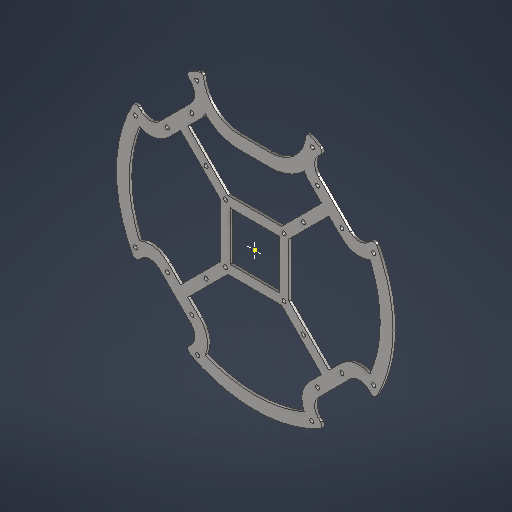
# Autodesk Inventor part: Mittelding mit IR Halterung
Saved by Autodesk Inventor 2025.3 (Build 293356000, 356)
## iProperties
Created: 2024-10-04
Part Number: Mittelding mit IR Halterung
Material: Generisch
Document SubType Name: Modeling
Designer: Mathimazierer
Density: 1 g/cm^3
Appearance: Halbpoliert
Author: Mathimazierer
Autodesk Inventor part; units mm, degrees
ref_plane "YZ Plane" through (0, 0, 0) normal (1, 0, 0) x (0, 1, 0)
ref_plane "XZ Plane" through (0, 0, 0) normal (0, 1, 0) x (-1, 0, 0)
ref_plane "XY Plane" through (0, 0, 0) normal (0, 0, 1) x (1, 0, 0)
sketch "Skizze1" plane through (0, 0, 0) normal (0, 1, 0) x (-1, 0, 0)
  circle A0 centre (48.7904, 67.8822) radius 1.6
  circle A1 centre (48.7904, -67.8823) radius 1.6
  circle A2 centre (-48.7904, -67.8822) radius 1.6
  circle A3 centre (-48.7904, 67.8823) radius 1.6
  circle A4 centre (67.8823, 48.7904) radius 1.6
  circle A5 centre (67.8822, -48.7904) radius 1.6
  circle A6 centre (-67.8823, -48.7904) radius 1.6
  circle A7 centre (-67.8822, 48.7904) radius 1.6
  arc A8 (42.6492, 98.6778) -> (39.8653, 97.0378) centre (41.8557, 96.8419) ccw
  arc A9 (12, 71.781) -> (39.8653, 97.0378) centre (12, 99.781) ccw
  line L0 (-12, 71.781) -> (12, 71.781)
  arc A10 (-39.8653, 97.0378) -> (-12, 71.781) centre (-12, 99.781) ccw
  arc A11 (-39.8653, 97.0378) -> (-42.6492, 98.6778) centre (-41.8557, 96.8419) ccw
  arc A12 (-42.6492, 98.6778) -> (-50.5184, 94.8902) centre (0, 0) ccw
  arc A13 (-50.5184, 94.8902) -> (-51.2299, 90.1208) centre (-49.1086, 92.2421) ccw
  line L1 (-49.4975, 88.3883) -> (-51.2299, 90.1208)
  arc A14 (-49.4975, 74.2462) -> (-49.4975, 88.3883) centre (-56.5685, 81.3173) ccw
  line L2 (-74.2462, 49.4975) -> (-49.4975, 74.2462)
  arc A15 (-88.3883, 49.4975) -> (-74.2462, 49.4975) centre (-81.3173, 56.5685) ccw
  line L3 (-90.1207, 51.2299) -> (-88.3883, 49.4975)
  arc A16 (-90.1207, 51.2299) -> (-94.8902, 50.5184) centre (-92.2421, 49.1086) ccw
  arc A17 (-94.8902, 50.5184) -> (-94.8902, -50.5184) centre (0, 0) ccw
  arc A18 (-94.8902, -50.5184) -> (-90.1208, -51.2299) centre (-92.2421, -49.1086) ccw
  line L4 (-88.3883, -49.4975) -> (-90.1208, -51.2299)
  arc A19 (-74.2462, -49.4975) -> (-88.3883, -49.4975) centre (-81.3173, -56.5685) ccw
  line L5 (-49.4975, -74.2462) -> (-74.2462, -49.4975)
  arc A20 (-49.4975, -88.3883) -> (-49.4975, -74.2462) centre (-56.5685, -81.3173) ccw
  line L6 (-51.2299, -90.1207) -> (-49.4975, -88.3883)
  arc A21 (-51.2299, -90.1207) -> (-50.5184, -94.8902) centre (-49.1086, -92.2421) ccw
  arc A22 (-50.5184, -94.8902) -> (50.5184, -94.8902) centre (0, 0) ccw
  arc A23 (50.5184, -94.8902) -> (51.2299, -90.1208) centre (49.1086, -92.2421) ccw
  line L7 (49.4975, -88.3883) -> (51.2299, -90.1208)
  arc A24 (49.4975, -74.2462) -> (49.4975, -88.3883) centre (56.5685, -81.3173) ccw
  line L8 (74.2462, -49.4975) -> (49.4975, -74.2462)
  arc A25 (88.3883, -49.4975) -> (74.2462, -49.4975) centre (81.3173, -56.5685) ccw
  line L9 (90.1207, -51.2299) -> (88.3883, -49.4975)
  arc A26 (90.1207, -51.2299) -> (94.8902, -50.5184) centre (92.2421, -49.1086) ccw
  arc A27 (94.8902, -50.5184) -> (94.8902, 50.5184) centre (0, 0) ccw
  arc A28 (94.8902, 50.5184) -> (90.1208, 51.2299) centre (92.2421, 49.1086) ccw
  line L10 (88.3883, 49.4975) -> (90.1208, 51.2299)
  arc A29 (74.2462, 49.4975) -> (88.3883, 49.4975) centre (81.3173, 56.5685) ccw
  line L11 (49.4975, 74.2462) -> (74.2462, 49.4975)
  arc A30 (49.4975, 88.3883) -> (49.4975, 74.2462) centre (56.5685, 81.3173) ccw
  line L12 (51.2299, 90.1207) -> (49.4975, 88.3883)
  arc A31 (51.2299, 90.1207) -> (50.5184, 94.8902) centre (49.1086, 92.2421) ccw
  arc A32 (50.5184, 94.8902) -> (42.6492, 98.6778) centre (0, 0) ccw
  line L13 (-107.5, 0) -> (-97.5, 0)
  circle A33 centre (0, 0) radius 97.5
  line L14 (0, 71.781) -> (0, 61.781)
  line L15 (-12, 99.781) -> (12, 99.781) construction
  line L16 (-12, 137.781) -> (12, 137.781)
  line L17 (12, 61.781) -> (-12, 61.781)
  arc A34 (-12, 137.781) -> (-12, 61.781) centre (-12, 99.781) ccw
  arc A35 (12, 61.781) -> (12, 137.781) centre (12, 99.781) ccw
  circle A36 centre (0, 0) radius 107.5
  line L18 (61.8718, 61.8718) -> (54.8008, 54.8008)
  line L19 (56.5685, 81.3173) -> (81.3173, 56.5685) construction
  line L20 (70.7107, 95.4594) -> (95.4594, 70.7107)
  line L21 (67.1751, 42.4264) -> (42.4264, 67.1751)
  arc A37 (70.7107, 95.4594) -> (42.4264, 67.1751) centre (56.5685, 81.3173) ccw
  arc A38 (67.1751, 42.4264) -> (95.4594, 70.7107) centre (81.3173, 56.5685) ccw
  line L22 (-95.4594, 70.7107) -> (-70.7107, 95.4594)
  arc A39 (-95.4594, 70.7107) -> (-67.1751, 42.4264) centre (-81.3173, 56.5685) ccw
  line L23 (-42.4264, 67.1751) -> (-67.1751, 42.4264)
  arc A40 (-42.4264, 67.1751) -> (-70.7107, 95.4594) centre (-56.5685, 81.3173) ccw
  line L24 (-70.7107, -95.4594) -> (-95.4594, -70.7107)
  arc A41 (-70.7107, -95.4594) -> (-42.4264, -67.1751) centre (-56.5685, -81.3173) ccw
  line L25 (-67.1751, -42.4264) -> (-42.4264, -67.1751)
  arc A42 (-67.1751, -42.4264) -> (-95.4594, -70.7107) centre (-81.3173, -56.5685) ccw
  line L26 (95.4594, -70.7107) -> (70.7107, -95.4594)
  arc A43 (95.4594, -70.7107) -> (67.1751, -42.4264) centre (81.3173, -56.5685) ccw
  line L27 (42.4264, -67.1751) -> (67.1751, -42.4264)
  arc A44 (42.4264, -67.1751) -> (70.7107, -95.4594) centre (56.5685, -81.3173) ccw
  point P0 (0, 0)
  point P1 (0, 99.781)
  point P2 (68.9429, 68.9429)
  point P3 (38.5642, 72.6085)
  point P4 (89.6293, 38.3776)
  point P5 (89.6293, -38.3776)
  point P6 (38.3776, -89.6293)
  point P7 (-38.3776, -89.6293)
  point P8 (-89.6293, -38.3776)
  point P9 (-89.6293, 38.3776)
  point P10 (-38.5642, 72.6085)
  dimension "d2" = 10
  dimension "d3" = 10
  dimension "d4" = 10
  dimension "d5" = 360
  constraints: 71 point on circle, 60 end point, 44 centre point, 8 tangent, 4 midpoint, 2 horizontal, 2 parallel, 1 coincident, 1 concentric, 1 vertical, 44 other
  measures "d2" distance of L13.start L13.end
  measures "d3" distance of L14.start L14.end
  measures "d4" distance of L18.start L18.end
extrude "Extrusion1" add sketch "Skizze1" along normal blind 2 contours A32 A37 A33 A9 A8 | A32 A35 A33 A37 | A11 A10 A33 A40 A12 | A33 A37 A35 L17 L14 L0 A9 | A32 A31 L12 A30 A33 A35 | A33 A35 A37 | A40 A33 A34 A12 | A10 L0 L14 L17 A34 A40 A33 | A33 A30 L11 L18 L21 A37 A35 | A34 A33 A14 L1 A13 A12 | A40 A34 A33 | A27 A38 A33 A29 L10 A28 | A34 A40 L23 A39 A33 A15 L2 A14 | A27 A43 A33 A38 | A33 A38 L21 L18 L11 A29 | A16 L3 A15 A33 A39 A17 | A39 A33 L13 A17 | A27 A26 L9 A25 A33 A43 | L13 A33 A42 A17 | A33 A25 L8 A24 A44 L27 A43 | A42 A33 A19 L4 A18 A17 | A22 A44 A33 A24 L7 A23 | A42 L25 A41 A33 A20 L5 A19 | A22 A41 A33 A44 | A21 L6 A20 A33 A41 A22
sketch "Skizze2" plane through (0, 0, 0) normal (0, -1, 0) x (1, 0, 0)
  line L0 (-12, 71.781) -> (12, 71.781)
  line L1 (0, 71.781) -> (-45, 71.781)
  line L2 (-45, 71.781) -> (-45, 90.181)
  circle A0 centre (-45, 91.781) radius 1.6
  circle A1 centre (45, 91.781) radius 1.6
  line L3 (-45, 91.781) -> (-43.4, 91.781)
  line L4 (43.4, 91.781) -> (45, 91.781)
  point P0 (0, 0)
  point P1 (0, 0)
  dimension "d12" = 3.2
  dimension "d8" = 45
  dimension "d9" = 20
  dimension "d10" = 90
  dimension "d11" = 3.2
  constraints: 10 end point, 3 perpendicular, 2 coincident, 2 point on circle, 1 centre point, 1 collinear, 1 horizontal alignment, 1 midpoint, 2 other
  measures "d8" distance of L1.start L1.end
  measures "d9" distance of L1.end L3.start
  measures "d10" distance of L3.start L4.end
  measures "d11" diameter of A0
extrude "Extrusion2" cut sketch "Skizze2" against normal blind 2
sketch "Skizze4" plane through (0, 0, 0) normal (0, -1, 0) x (1, 0, 0)
  arc A0 (-89.6293, 38.3776) -> (-67.1751, 42.4264) centre (-81.3173, 56.5685) ccw projected
  line L0 (-89.6293, 38.3776) -> (-92.6293, 38.3776)
  line L1 (-92.6293, 38.3776) -> (-92.6293, 44.3776)
  circle A1 centre (-92.6293, 44.3776) radius 1.6
  line L2 (0, 0) -> (0, 25.0605)
  circle A2 centre (92.6293, 44.3776) radius 1.6
  line L3 (0, 0) -> (24.0144, 0)
  circle A3 centre (-92.6293, -44.3776) radius 1.6
  circle A4 centre (92.6293, -44.3776) radius 1.6
  circle A5 centre (-44.3776, -92.6293) radius 1.6
  circle A6 centre (44.3776, -92.6293) radius 1.6
  point P0 (0, 0)
  dimension "d15" = 3
  dimension "d16" = 6
  dimension "d17" = 3.2
  dimension "d18" = 3.2
  constraints: 8 end point, 6 centre point, 3 symmetric about line, 2 horizontal, 1 coincident, 1 perpendicular, 1 vertical, 3 other
  measures "d15" distance of L0.start L0.end
  measures "d16" distance of L0.end L1.end
  measures "d17" diameter of A1
  measures "d18" diameter of A5
extrude "Extrusion3" cut sketch "Skizze4" against normal blind 3.2
sketch "Skizze5" plane through (0, 0, 0) normal (0, -1, 0) x (1, 0, 0)
  line L0 (-42.4264, 67.1751) -> (-67.1751, 42.4264) projected
  line L1 (-54.8008, 54.8008) -> (-14.8008, 54.8008) construction
  line L2 (-54.8008, 54.8008) -> (-26.5165, 26.5165)
  line L3 (-54.8008, -54.8008) -> (-26.5165, -26.5165)
  line L4 (54.8008, -54.8008) -> (26.5165, -26.5165)
  line L5 (54.8008, 54.8008) -> (26.5165, 26.5165)
  line L6 (-26.5165, 26.5165) -> (-26.5165, -26.5165)
  line L7 (26.5165, -26.5165) -> (-26.5165, -26.5165)
  line L8 (26.5165, -26.5165) -> (26.5165, 26.5165)
  line L9 (-26.5165, 26.5165) -> (26.5165, 26.5165)
  line L10 (-54.8008, 54.8008) -> (-57.6292, 51.9723)
  line L11 (-57.6292, 51.9723) -> (-51.9724, 57.6292)
  line L12 (-51.9724, 57.6292) -> (-20.8597, 26.5165)
  line L13 (-57.6292, 51.9723) -> (-26.5165, 20.8596)
  line L14 (-57.6292, -51.9724) -> (-26.5165, -20.8597)
  line L15 (-51.9723, -57.6292) -> (-20.8596, -26.5165)
  line L16 (51.9724, -57.6292) -> (20.8597, -26.5165)
  line L17 (57.6292, -51.9723) -> (26.5165, -20.8596)
  line L18 (57.6292, 51.9724) -> (26.5165, 20.8597)
  line L19 (51.9723, 57.6292) -> (20.8596, 26.5165)
  line L20 (51.9723, 57.6292) -> (57.6292, 51.9724)
  line L21 (51.9724, -57.6292) -> (57.6292, -51.9723)
  line L22 (-57.6292, -51.9724) -> (-51.9723, -57.6292)
  line L23 (-67.1751, -42.4264) -> (-42.4264, -67.1751) projected
  line L24 (-26.5165, 26.5165) -> (-26.5165, 19.0165)
  line L25 (-26.5165, 19.0165) -> (-19.0165, 19.0165)
  line L26 (26.5165, -26.5165) -> (19.0165, -26.5165)
  line L27 (19.0165, -26.5165) -> (19.0165, -19.0165)
  line L28 (-19.0165, 19.0165) -> (19.0165, 19.0165)
  line L29 (19.0165, 19.0165) -> (19.0165, -19.0165)
  line L30 (19.0165, -19.0165) -> (-19.0165, -19.0165)
  line L31 (-19.0165, -19.0165) -> (-19.0165, 19.0165)
  circle A0 centre (-22.7665, 22.7665) radius 1.6
  circle A1 centre (22.7665, 22.7665) radius 1.6
  circle A2 centre (-22.7665, -22.7665) radius 1.6
  circle A3 centre (22.7665, -22.7665) radius 1.6
  line L32 (-26.5165, 20.8596) -> (-40.6586, 35.0018)
  line L33 (-40.6586, 35.0018) -> (-37.8302, 37.8302)
  circle A4 centre (-37.8302, 37.8302) radius 1.65
  circle A5 centre (-37.8302, -37.8302) radius 1.65
  circle A6 centre (37.8302, -37.8302) radius 1.65
  circle A7 centre (37.8302, 37.8302) radius 1.65
  point P0 (0, 0)
  point P1 (-26.5165, -20.8597)
  point P2 (20.8597, -26.5165)
  point P3 (26.5165, 20.8597)
  dimension "d23" = 40
  dimension "d26" = 360
  dimension "d28" = 4
  dimension "d29" = 8
  dimension "d32" = 360
  dimension "d34" = 7.5
  dimension "d35" = 7.5
  dimension "d36" = 7.5
  dimension "d37" = 7.5
  dimension "d38" = 3.2
  dimension "d39" = 3.2
  dimension "d40" = 3.2
  dimension "d41" = 3.2
  dimension "d44" = 20
  dimension "d45" = 3.3
  dimension "d48" = 360
  constraints: 64 end point, 10 perpendicular, 8 centre point, 8 point on line, 3 parallel, 2 horizontal, 1 coincident, 1 collinear, 1 midpoint, 1 vertical, 47 other
  measures "d23" distance of L1.start L2.end
  measures "d28" distance of L1.start L10.end
  measures "d29" distance of L10.end L11.end
  measures "d34" distance of L2.end L24.end
  measures "d35" distance of L24.end L25.end
  measures "d36" distance of L4.end L26.end
  measures "d37" distance of L26.end L27.end
  measures "d38" diameter of A0
  measures "d39" diameter of A1
  measures "d40" diameter of A2
  measures "d41" diameter of A3
  measures "d44" distance of L13.end L32.end
  measures "d45" diameter of A4
extrude "Extrusion4" add sketch "Skizze5" against normal blind 2 contours L12 L9 L2 A4 L0 | L2 A4 L33 L13 L0 | L9 L8 L7 L27 L29 L28 L25 L6 | A4 L2 | L2 L33 A4 | L6 L13 L33 A4 L2 | L19 L20 L5 A7 L9 | L2 A4 L33 | L5 A7 L20 L18 L8 | L25 L31 L30 L27 L7 L6 | A7 L5 | L5 A7 | L6 L3 A5 L22 L14 | L17 L21 L4 A6 L8 | L7 L15 L22 L3 A5 | L4 A6 L21 L16 L7 | A5 L3 | L3 A5 | A6 L4 | L4 A6
sketch "Skizze6" plane through (0, 2, 0) normal (0, 1, 0) x (1, 0, 0)
  line L0 (-51.9723, 57.6292) -> (-42.4264, 67.1751) projected
  arc A0 (-42.4264, 67.1751) -> (-38.3776, 89.6293) centre (-56.5685, 81.3173) ccw projected
  arc A1 (38.3776, 89.6293) -> (-38.3776, 89.6293) centre (0, 0) ccw projected
  arc A2 (38.3776, 89.6293) -> (42.4264, 67.1751) centre (56.5685, 81.3173) ccw projected
  line L1 (42.4264, 67.1751) -> (51.9724, 57.6292) projected
  line L2 (51.9724, 57.6292) -> (20.8597, 26.5165) projected
  line L3 (20.8597, 26.5165) -> (-20.8596, 26.5165) projected
  line L4 (-20.8596, 26.5165) -> (-51.9723, 57.6292) projected
  line L5 (57.6292, 51.9723) -> (67.1751, 42.4264) projected
  arc A3 (67.1751, 42.4264) -> (89.6293, 38.3776) centre (81.3173, 56.5685) ccw projected
  arc A4 (89.6293, -38.3776) -> (89.6293, 38.3776) centre (0, 0) ccw projected
  arc A5 (89.6293, -38.3776) -> (67.1751, -42.4264) centre (81.3173, -56.5685) ccw projected
  line L6 (67.1751, -42.4264) -> (57.6292, -51.9724) projected
  line L7 (57.6292, -51.9724) -> (26.5165, -20.8597) projected
  line L8 (26.5165, -20.8597) -> (26.5165, 20.8596) projected
  line L9 (26.5165, 20.8596) -> (57.6292, 51.9723) projected
  line L10 (51.9723, -57.6292) -> (42.4264, -67.1751) projected
  arc A6 (42.4264, -67.1751) -> (38.5642, -72.6085) centre (56.5685, -81.3173) ccw projected
  arc A7 (38.5642, -72.6085) -> (12, -61.781) centre (12, -99.781) ccw projected
  line L11 (12, -61.781) -> (-12, -61.781) projected
  arc A8 (-12, -61.781) -> (-38.5642, -72.6085) centre (-12, -99.781) ccw projected
  arc A9 (-38.5642, -72.6085) -> (-42.4264, -67.1751) centre (-56.5685, -81.3173) ccw projected
  line L12 (-42.4264, -67.1751) -> (-51.9724, -57.6292) projected
  line L13 (-51.9724, -57.6292) -> (-20.8597, -26.5165) projected
  line L14 (-20.8597, -26.5165) -> (20.8596, -26.5165) projected
  line L15 (20.8596, -26.5165) -> (51.9723, -57.6292) projected
  circle A10 centre (-22.7665, -22.7665) radius 1.6 projected
  circle A11 centre (22.7665, -22.7665) radius 1.6 projected
  circle A12 centre (22.7665, 22.7665) radius 1.6 projected
  circle A13 centre (-22.7665, 22.7665) radius 1.6 projected
  line L16 (19.0165, -19.0165) -> (-19.0165, -19.0165) projected
  line L17 (-19.0165, -19.0165) -> (-19.0165, 19.0165) projected
  line L18 (-19.0165, 19.0165) -> (19.0165, 19.0165) projected
  line L19 (19.0165, 19.0165) -> (19.0165, -19.0165) projected
  circle A14 centre (-44.3776, 92.6293) radius 1.6 projected
  circle A15 centre (92.6293, -44.3776) radius 1.6 projected
  circle A16 centre (-92.6293, 44.3776) radius 1.6 projected
  circle A17 centre (44.3776, 92.6293) radius 1.6 projected
  circle A18 centre (92.6293, 44.3776) radius 1.6 projected
  circle A19 centre (-92.6293, -44.3776) radius 1.6 projected
  circle A20 centre (45, -91.781) radius 1.6 projected
  circle A21 centre (-45, -91.781) radius 1.6 projected
  arc A22 (39.8653, -97.0378) -> (12, -71.781) centre (12, -99.781) ccw projected
  arc A23 (39.8653, -97.0378) -> (42.6492, -98.6778) centre (41.8557, -96.8419) ccw projected
  arc A24 (42.6492, -98.6778) -> (50.5184, -94.8902) centre (0, 0) ccw projected
  arc A25 (50.5184, -94.8902) -> (51.2299, -90.1208) centre (49.1086, -92.2421) ccw projected
  line L20 (51.2299, -90.1208) -> (49.4975, -88.3883) projected
  arc A26 (49.4975, -74.2462) -> (49.4975, -88.3883) centre (56.5685, -81.3173) ccw projected
  line L21 (49.4975, -74.2462) -> (74.2462, -49.4975) projected
  arc A27 (88.3883, -49.4975) -> (74.2462, -49.4975) centre (81.3173, -56.5685) ccw projected
  line L22 (88.3883, -49.4975) -> (90.1207, -51.2299) projected
  arc A28 (90.1207, -51.2299) -> (94.8902, -50.5184) centre (92.2421, -49.1086) ccw projected
  arc A29 (94.8902, -50.5184) -> (94.8902, 50.5184) centre (0, 0) ccw projected
  arc A30 (94.8902, 50.5184) -> (90.1208, 51.2299) centre (92.2421, 49.1086) ccw projected
  line L23 (90.1208, 51.2299) -> (88.3883, 49.4975) projected
  arc A31 (74.2462, 49.4975) -> (88.3883, 49.4975) centre (81.3173, 56.5685) ccw projected
  line L24 (74.2462, 49.4975) -> (49.4975, 74.2462) projected
  arc A32 (49.4975, 88.3883) -> (49.4975, 74.2462) centre (56.5685, 81.3173) ccw projected
  line L25 (49.4975, 88.3883) -> (51.2299, 90.1207) projected
  arc A33 (51.2299, 90.1207) -> (50.5184, 94.8902) centre (49.1086, 92.2421) ccw projected
  arc A34 (50.5184, 94.8902) -> (-50.5184, 94.8902) centre (0, 0) ccw projected
  arc A35 (-50.5184, 94.8902) -> (-51.2299, 90.1208) centre (-49.1086, 92.2421) ccw projected
  line L26 (-51.2299, 90.1208) -> (-49.4975, 88.3883) projected
  arc A36 (-49.4975, 74.2462) -> (-49.4975, 88.3883) centre (-56.5685, 81.3173) ccw projected
  line L27 (-49.4975, 74.2462) -> (-74.2462, 49.4975) projected
  arc A37 (-88.3883, 49.4975) -> (-74.2462, 49.4975) centre (-81.3173, 56.5685) ccw projected
  line L28 (-88.3883, 49.4975) -> (-90.1207, 51.2299) projected
  arc A38 (-90.1207, 51.2299) -> (-94.8902, 50.5184) centre (-92.2421, 49.1086) ccw projected
  arc A39 (-94.8902, 50.5184) -> (-94.8902, -50.5184) centre (0, 0) ccw projected
  arc A40 (-94.8902, -50.5184) -> (-90.1208, -51.2299) centre (-92.2421, -49.1086) ccw projected
  line L29 (-90.1208, -51.2299) -> (-88.3883, -49.4975) projected
  arc A41 (-74.2462, -49.4975) -> (-88.3883, -49.4975) centre (-81.3173, -56.5685) ccw projected
  line L30 (-74.2462, -49.4975) -> (-49.4975, -74.2462) projected
  arc A42 (-49.4975, -88.3883) -> (-49.4975, -74.2462) centre (-56.5685, -81.3173) ccw projected
  line L31 (-49.4975, -88.3883) -> (-51.2299, -90.1207) projected
  arc A43 (-51.2299, -90.1207) -> (-50.5184, -94.8902) centre (-49.1086, -92.2421) ccw projected
  arc A44 (-50.5184, -94.8902) -> (-42.6492, -98.6778) centre (0, 0) ccw projected
  arc A45 (-42.6492, -98.6778) -> (-39.8653, -97.0378) centre (-41.8557, -96.8419) ccw projected
  arc A46 (-12, -71.781) -> (-39.8653, -97.0378) centre (-12, -99.781) ccw projected
  line L32 (-12, -71.781) -> (12, -71.781) projected
  line L33 (-57.6292, 51.9724) -> (-26.5165, 20.8597) projected
  line L34 (-26.5165, 20.8597) -> (-26.5165, -20.8596) projected
  line L35 (-26.5165, -20.8596) -> (-57.6292, -51.9723) projected
  line L36 (-57.6292, -51.9723) -> (-67.1751, -42.4264) projected
  arc A47 (-67.1751, -42.4264) -> (-89.6293, -38.3776) centre (-81.3173, -56.5685) ccw projected
  arc A48 (-89.6293, 38.3776) -> (-89.6293, -38.3776) centre (0, 0) ccw projected
  arc A49 (-89.6293, 38.3776) -> (-67.1751, 42.4264) centre (-81.3173, 56.5685) ccw projected
  line L37 (-67.1751, 42.4264) -> (-57.6292, 51.9724) projected
  circle A50 centre (-48.7904, -67.8822) radius 1.6 projected
  circle A51 centre (48.7904, -67.8823) radius 1.6 projected
  circle A52 centre (67.8822, -48.7904) radius 1.6 projected
  circle A53 centre (-67.8823, -48.7904) radius 1.6 projected
  circle A54 centre (67.8823, 48.7904) radius 1.6 projected
  circle A55 centre (48.7904, 67.8822) radius 1.6 projected
  circle A56 centre (-48.7904, 67.8823) radius 1.6 projected
  circle A57 centre (-67.8822, 48.7904) radius 1.6 projected
sketch "Skizze8" plane through (0, 0, 0) normal (0, -1, 0) x (1, 0, 0)
  line L0 (-314.1721, 98.2713) -> (-338.9208, 73.5225)
  line L1 (-326.5464, 85.8969) -> (-286.5464, 85.8969) construction
  line L2 (-326.5464, 85.8969) -> (-298.2622, 57.6126)
  line L3 (-326.5464, -23.7046) -> (-298.2622, 4.5796)
  line L4 (-216.9449, -23.7046) -> (-245.2292, 4.5796)
  line L5 (-216.9449, 85.8969) -> (-245.2292, 57.6126)
  line L6 (-298.2622, 57.6126) -> (-298.2622, 4.5796)
  line L7 (-245.2292, 4.5796) -> (-298.2622, 4.5796)
  line L8 (-245.2292, 4.5796) -> (-245.2292, 57.6126)
  line L9 (-298.2622, 57.6126) -> (-245.2292, 57.6126)
  line L10 (-326.5464, 85.8969) -> (-329.3749, 83.0685)
  line L11 (-329.3749, 83.0685) -> (-323.718, 88.7253)
  line L12 (-323.718, 88.7253) -> (-292.6053, 57.6126)
  line L13 (-329.3749, 83.0685) -> (-298.2622, 51.9558)
  line L14 (-329.3749, -20.8762) -> (-298.2622, 10.2365)
  line L15 (-323.718, -26.5331) -> (-292.6053, 4.5796)
  line L16 (-219.7733, -26.5331) -> (-250.886, 4.5796)
  line L17 (-214.1165, -20.8762) -> (-245.2292, 10.2365)
  line L18 (-214.1165, 83.0685) -> (-245.2292, 51.9558)
  line L19 (-219.7733, 88.7253) -> (-250.886, 57.6126)
  line L20 (-329.3749, -20.8762) -> (-323.718, -26.5331)
  line L21 (-338.9208, -11.3303) -> (-314.1721, -36.079)
  line L22 (-298.2622, 57.6126) -> (-298.2622, 50.1126)
  line L23 (-298.2622, 50.1126) -> (-290.7622, 50.1126)
  line L24 (-245.2292, 4.5796) -> (-252.7292, 4.5796)
  line L25 (-252.7292, 4.5796) -> (-252.7292, 12.0796)
  line L26 (-290.7622, 50.1126) -> (-252.7292, 50.1126)
  line L27 (-252.7292, 50.1126) -> (-252.7292, 12.0796)
  line L28 (-252.7292, 12.0796) -> (-290.7622, 12.0796)
  line L29 (-290.7622, 12.0796) -> (-290.7622, 50.1126)
  circle A0 centre (-294.5122, 53.8626) radius 1.6
  circle A1 centre (-248.9792, 53.8626) radius 1.6
  circle A2 centre (-294.5122, 8.3296) radius 1.6
  circle A3 centre (-248.9792, 8.3296) radius 1.6
  line L30 (-298.2622, 51.9558) -> (-312.4043, 66.0979)
  line L31 (-312.4043, 66.0979) -> (-309.5759, 68.9264)
  circle A4 centre (-309.5759, 68.9264) radius 1.65
  circle A5 centre (-309.5759, -6.7341) radius 1.65
  circle A6 centre (-233.9155, -6.7341) radius 1.65
  circle A7 centre (-233.9155, 68.9264) radius 1.65
  line L32 (-26.5165, 20.8596) -> (-26.5165, -20.8597) projected
  line L33 (-26.5165, 20.8596) -> (-40.6586, 35.0018)
  line L34 (-57.6292, 51.9723) -> (-26.5165, 20.8596) projected
  line L35 (-40.6586, 35.0018) -> (-35.0018, 40.6586)
  line L36 (-51.9724, 57.6292) -> (-20.8597, 26.5165) projected
  circle A8 centre (-37.8302, 37.8302) radius 1.65
  circle A9 centre (-37.8302, -37.8302) radius 1.65
  circle A10 centre (37.8302, -37.8302) radius 1.65
  circle A11 centre (37.8302, 37.8302) radius 1.65
  point P0 (0, 0)
  point P1 (-271.7457, 31.0961)
  point P2 (-298.2622, 10.2365)
  point P3 (-292.6053, 4.5796)
  point P4 (-250.886, 4.5796)
  point P5 (-245.2292, 10.2365)
  point P6 (-245.2292, 51.9558)
  point P7 (-250.886, 57.6126)
  dimension "d56" = 40
  dimension "d57" = 360
  dimension "d58" = 4
  dimension "d59" = 8
  dimension "d60" = 360
  dimension "d61" = 7.5
  dimension "d62" = 7.5
  dimension "d63" = 7.5
  dimension "d64" = 7.5
  dimension "d65" = 3.2
  dimension "d66" = 3.2
  dimension "d67" = 3.2
  dimension "d68" = 3.2
  dimension "d69" = 20
  dimension "d70" = 3.3
  dimension "d71" = 360
  dimension "d72" = 20
  dimension "d73" = 3.3
  dimension "d76" = 360
  constraints: 68 end point, 12 centre point, 10 point on line, 9 perpendicular, 3 parallel, 2 coincident, 2 horizontal, 2 midpoint, 1 collinear, 1 vertical, 56 other
  measures "d56" distance of L1.start L2.end
  measures "d58" distance of L1.start L10.end
  measures "d59" distance of L10.end L11.end
  measures "d61" distance of L2.end L22.end
  measures "d62" distance of L22.end L23.end
  measures "d63" distance of L4.end L24.end
  measures "d64" distance of L24.end L25.end
  measures "d65" diameter of A0
  measures "d66" diameter of A1
  measures "d67" diameter of A2
  measures "d68" diameter of A3
  measures "d69" distance of L13.end L30.end
  measures "d70" diameter of A4
  measures "d72" distance of L32.start L33.end
  measures "d73" diameter of A8
extrude "Extrusion5" cut sketch "Skizze8" against normal blind 10 contours A8 L35 | L35 A8 | A9 | A10 | A11
sketch "Skizze9" plane through (0, 0, 0) normal (0, -1, 0) x (1, 0, 0)
  circle A0 centre (-14.732, 5.2251) radius 1.4
  circle A1 centre (14.732, 5.2251) radius 1.4
  circle A2 centre (0, 0) radius 4.85
  circle A3 centre (-22.7665, 22.7665) radius 1.6 projected
  circle A4 centre (-22.7665, 22.7665) radius 1.6
  circle A5 centre (22.7665, 22.7665) radius 1.6 projected
  circle A6 centre (22.7665, 22.7665) radius 1.6
  circle A7 centre (22.7665, -22.7665) radius 1.6 projected
  circle A8 centre (22.7665, -22.7665) radius 1.6
  circle A9 centre (-22.7665, -22.7665) radius 1.6 projected
  circle A10 centre (-22.7665, -22.7665) radius 1.6
  line L0 (-22.7665, 22.7665) -> (-25.7665, 22.7665)
  line L1 (-25.7665, 22.7665) -> (-25.7665, 25.7665)
  line L2 (-22.7665, 22.7665) -> (-22.7665, 19.7665)
  line L3 (-22.7665, 19.7665) -> (-19.7665, 19.7665)
  line L4 (22.7665, -22.7665) -> (25.7665, -22.7665)
  line L5 (25.7665, -22.7665) -> (25.7665, -25.7665)
  line L6 (22.7665, -22.7665) -> (22.7665, -19.7665)
  line L7 (22.7665, -19.7665) -> (19.7665, -19.7665)
  line L8 (-25.7665, 25.7665) -> (25.7665, 25.7665)
  line L9 (25.7665, 25.7665) -> (25.7665, -25.7665)
  line L10 (25.7665, -25.7665) -> (-25.7665, -25.7665)
  line L11 (-25.7665, -25.7665) -> (-25.7665, 25.7665)
  line L12 (19.7665, -19.7665) -> (-19.7665, -19.7665)
  line L13 (-19.7665, -19.7665) -> (-19.7665, 19.7665)
  line L14 (-19.7665, 19.7665) -> (19.7665, 19.7665)
  line L15 (19.7665, 19.7665) -> (19.7665, -19.7665)
  line L16 (-14.732, 5.2251) -> (-14.732, 3.2251)
  line L17 (-14.732, 3.2251) -> (-14.732, 7.2251)
  line L18 (-14.732, 7.2251) -> (-19.7665, 7.2251)
  line L19 (-14.732, 3.2251) -> (-19.7665, 3.2251)
  circle A11 centre (-14.732, 5.2251) radius 2
  line L20 (0, 4.85) -> (0, 5.85)
  circle A12 centre (14.732, 5.2251) radius 1.4
  line L21 (14.732, 7.2251) -> (19.7665, 7.2251)
  line L22 (14.732, 3.2251) -> (19.7665, 3.2251)
  circle A13 centre (14.732, 5.2251) radius 2
  dimension "d84" = 3
  dimension "d85" = 3
  dimension "d86" = 3
  dimension "d88" = 3
  dimension "d89" = 3
  dimension "d90" = 3
  dimension "d91" = 3
  dimension "d92" = 3
  dimension "d93" = 2
  dimension "d94" = 4
  dimension "d95" = 1
  constraints: 46 end point, 7 centre point, 7 perpendicular, 6 coincident, 6 symmetric about line, 5 horizontal, 5 vertical, 4 parallel, 3 point on line, 3 vertical alignment, 7 other
  measures "d84" distance of L0.start L0.end
  measures "d85" distance of L0.end L1.end
  measures "d86" distance of L0.start L2.end
  measures "d88" distance of L2.end L3.end
  measures "d89" distance of L4.start L4.end
  measures "d90" distance of L4.end L5.end
  measures "d91" distance of L4.start L6.end
  measures "d92" distance of L6.end L7.end
  measures "d93" distance of L16.start L16.end
  measures "d94" distance of L16.end L17.end
  measures "d95" distance of L20.start L20.end
fillet "Rundung1" radius 2 2 edges at (20.8597, 1, -26.5165) (-20.8596, 1, -26.5165)
sketch "Skizze14" plane through (0, 0, 0) normal (0, -1, 0) x (1, 0, 0)
  point P0 (0, 0)
  point P1 (0, 0)
  constraints: 1 coincident
equation "\"d19\" = d18"
